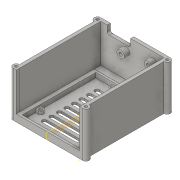
# Autodesk Inventor part: 11 electronics case
Saved by Autodesk Inventor 2016 (Build 200138000, 138)
## iProperties
Created: 2019-09-12
Part Number: 11 electronics case
Material: Generic
Document SubType Name: Modeling
Designer: mrbeh
Density: 1 g/cm^3
Appearance: Default
Author: mrbeh
Autodesk Inventor part; units mm, degrees
ref_plane "YZ Plane" through (0, 0, 0) normal (1, 0, 0) x (0, 1, 0)
ref_plane "XZ Plane" through (0, 0, 0) normal (0, 1, 0) x (-1, 0, 0)
ref_plane "XY Plane" through (0, 0, 0) normal (0, 0, 1) x (1, 0, 0)
sketch "Sketch1" plane through (0, 0, 0) normal (0, 1, 0) x (-1, 0, 0)
  line L0 (0, 0) -> (65, 0)
  line L1 (65, 0) -> (65, -85)
  line L2 (65, -85) -> (0, -85)
  line L3 (0, -85) -> (0, 0)
  dimension "d0" = 65
  dimension "d1" = 85
  constraints: 8 end point, 2 parallel, 1 horizontal, 1 perpendicular
  measures "d0" distance of L1.end L2.end
  measures "d1" distance of L0.end L1.end
extrude "Extrusion1" add sketch "Sketch1" along normal blind 2
sketch "Sketch2" plane through (0, 2, 0) normal (0, 1, 0) x (1, 0, 0)
  line L0 (-5.3227, 5.2279) -> (-58.5227, 5.2279)
  line L1 (-58.5227, 5.2279) -> (-58.5227, 73.9279)
  line L2 (-58.5227, 73.9279) -> (-5.3227, 73.9279)
  line L3 (-5.3227, 73.9279) -> (-5.3227, 5.2279)
  line L4 (-60.5227, 75.9279) -> (-60.5227, 3.2279)
  line L5 (-60.5227, 3.2279) -> (-3.3227, 3.2279)
  line L6 (-3.3227, 3.2279) -> (-3.3227, 75.9279)
  line L7 (-3.3227, 75.9279) -> (-60.5227, 75.9279)
  point P0 (0, 0)
  dimension "d4" = 53.2
  dimension "d5" = 68.7
  dimension "d6" = 2
  constraints: 16 end point, 4 parallel, 2 perpendicular, 1 horizontal, 3 other
  measures "d4" distance of L1.end L2.end
  measures "d5" distance of L0.end L1.end
  measures "d6" distance between parallel lines of L1 L4
extrude "Extrusion2" add sketch "Sketch2" along normal blind 5
ref_plane "Work Plane1" through (-31.9227, 2, -73.9279) normal (1, 0, 0) x (0, 0, -1)
sketch "Sketch4" plane through (0, 2, 0) normal (0, 1, 0) x (1, 0, 0)
  arc A0 (-56.0227, 17.7279) -> (-56.0227, 22.7279) centre (-56.0227, 20.2279) ccw
  line L0 (-58.5227, 5.2279) -> (-58.5227, 73.9279) projected
  line L1 (-56.0227, 17.7279) -> (-58.5227, 17.7279)
  line L2 (-58.5227, 17.7279) -> (-58.5227, 22.7279)
  line L3 (-58.5227, 22.7279) -> (-56.0227, 22.7279)
  point P0 (0, 0)
  dimension "d17" = 5
  constraints: 6 end point, 2 point on circle, 1 centre point, 1 horizontal, 1 parallel, 1 perpendicular, 1 point on line
  measures "d17" diameter of A0
extrude "Extrusion4" add sketch "Sketch4" along normal blind 3
sketch "Sketch5" plane through (0, 5, 0) normal (0, 1, 0) x (1, 0, 0)
  arc A0 (-56.0227, 17.7279) -> (-56.0227, 22.7279) centre (-56.0227, 20.2279) ccw projected
  circle A1 centre (-56.0227, 20.2279) radius 1.6
  point P0 (0, 0)
  dimension "d20" = 3.2
  constraints: 1 centre point, 1 coincident
  measures "d20" diameter of A1
extrude "Extrusion5" cut sketch "Sketch5" against normal blind 10
sketch "Sketch6" plane through (0, 2, 0) normal (0, 1, 0) x (1, 0, 0)
  line L0 (-5.3227, 73.9279) -> (-58.5227, 73.9279) projected
  line L1 (-5.3227, 73.9279) -> (-12.3227, 73.9279)
  line L2 (-5.3227, 71.4279) -> (-5.3227, 73.9279)
  arc A0 (-14.8227, 71.4279) -> (-9.8227, 71.4279) centre (-12.3227, 71.4279) ccw
  line L3 (-9.8227, 71.4279) -> (-9.8227, 73.9279)
  line L4 (-9.8227, 73.9279) -> (-14.8227, 73.9279)
  line L5 (-14.8227, 73.9279) -> (-14.8227, 71.4279)
  point P0 (0, 0)
  constraints: 10 end point, 2 point on circle, 1 centre point, 1 horizontal, 1 midpoint, 1 parallel, 1 point on line
extrude "Extrusion6" add sketch "Sketch6" along normal blind 3
sketch "Sketch7" plane through (0, 5, 0) normal (0, 1, 0) x (1, 0, 0)
  arc A0 (-14.8227, 71.4279) -> (-9.8227, 71.4279) centre (-12.3227, 71.4279) ccw projected
  circle A1 centre (-12.3227, 71.4279) radius 1.6
  point P0 (0, 0)
  dimension "d28" = 3.2
  constraints: 1 centre point, 1 coincident
  measures "d28" diameter of A1
extrude "Extrusion7" cut sketch "Sketch7" against normal blind 10
sketch "Sketch8" plane through (0, 2, 0) normal (0, 1, 0) x (1, 0, 0)
  line L0 (-5.3227, 5.2279) -> (-5.3227, 73.9279) projected
  line L1 (-5.3227, 73.9279) -> (-40.3227, 73.9279)
  line L2 (-5.3227, 71.4279) -> (-5.3227, 73.9279)
  arc A0 (-42.8227, 71.4279) -> (-37.8227, 71.4279) centre (-40.3227, 71.4279) ccw
  line L3 (-37.8227, 71.4279) -> (-37.8227, 73.9279)
  line L4 (-37.8227, 73.9279) -> (-42.8227, 73.9279)
  line L5 (-42.8227, 73.9279) -> (-42.8227, 71.4279)
  point P0 (0, 0)
  constraints: 10 end point, 2 point on circle, 1 centre point, 1 horizontal, 1 midpoint, 1 parallel, 1 point on line
extrude "Extrusion8" add sketch "Sketch8" along normal blind 3
sketch "Sketch9" plane through (0, 5, 0) normal (0, 1, 0) x (1, 0, 0)
  arc A0 (-42.8227, 71.4279) -> (-37.8227, 71.4279) centre (-40.3227, 71.4279) ccw projected
  circle A1 centre (-40.3227, 71.4279) radius 1.6
  point P0 (0, 0)
  dimension "d35" = 3.2
  constraints: 1 centre point, 1 coincident
  measures "d35" diameter of A1
extrude "Extrusion9" cut sketch "Sketch9" against normal blind 10
sketch "Sketch10" plane through (0, 2, 0) normal (0, 1, 0) x (1, 0, 0)
  line L0 (-5.3227, 5.2279) -> (-5.3227, 73.9279) projected
  line L1 (-5.3227, 19.2279) -> (-5.3227, 5.2279)
  arc A0 (-7.8227, 21.7279) -> (-7.8227, 16.7279) centre (-7.8227, 19.2279) ccw
  line L2 (-7.8227, 16.7279) -> (-5.3227, 16.7279)
  line L3 (-5.3227, 16.7279) -> (-5.3227, 21.7279)
  line L4 (-5.3227, 21.7279) -> (-7.8227, 21.7279)
  point P0 (0, 0)
  dimension "d40" = 5
  constraints: 8 end point, 2 point on circle, 1 centre point, 1 horizontal, 1 midpoint, 1 parallel, 1 perpendicular, 1 point on line
  measures "d40" diameter of A0
extrude "Extrusion10" add sketch "Sketch10" along normal blind 3
sketch "Sketch11" plane through (0, 5, 0) normal (0, 1, 0) x (1, 0, 0)
  arc A0 (-7.8227, 21.7279) -> (-7.8227, 16.7279) centre (-7.8227, 19.2279) ccw projected
  circle A1 centre (-7.8227, 19.2279) radius 1.6
  point P0 (0, 0)
  dimension "d43" = 3.2
  constraints: 1 centre point, 1 coincident
  measures "d43" diameter of A1
extrude "Extrusion11" cut sketch "Sketch11" against normal blind 10
sketch "Sketch12" plane through (0, 2, 0) normal (0, 1, 0) x (1, 0, 0)
  line L0 (-49.6328, 13.0575) -> (-14.6328, 13.0575)
  line L1 (-14.6328, 13.0575) -> (-14.6328, 17.0575)
  line L2 (-14.6328, 17.0575) -> (-49.6328, 17.0575)
  line L3 (-49.6328, 17.0575) -> (-49.6328, 13.0575)
  point P0 (0, 0)
  dimension "d46" = 35
  dimension "d47" = 4
  constraints: 8 end point, 2 parallel, 1 horizontal, 1 perpendicular
  measures "d46" distance of L2.end L1.end
  measures "d47" distance of L1.end L0.end
extrude "Extrusion12" cut sketch "Sketch12" against normal blind 10
fillet "Fillet1" radius 2 4 edges at (-49.6328, 1, -13.0575) (-49.6328, 1, -17.0575) (-14.6328, 1, -13.0575) (-14.6328, 1, -17.0575)
pattern_linear "Rectangular Pattern1" count 8 spacing 7 along (0, 0, -1) of "Extrusion12"
pattern_linear "Rectangular Pattern2" count 8 spacing 7 along (0, 0, -1) of "Fillet1"
sketch "Sketch13" plane through (0, 7, 0) normal (0, 1, 0) x (1, 0, 0)
  line L0 (4.8571, -9.3103) -> (-69.8772, -9.3103)
  line L1 (-69.8772, -9.3103) -> (-69.8772, 93.3248)
  line L2 (-69.8772, 93.3248) -> (4.8571, 93.3248)
  line L3 (4.8571, 93.3248) -> (4.8571, -9.3103)
  point P0 (0, 0)
  constraints: 8 end point, 2 parallel, 1 horizontal, 1 perpendicular
extrude "Extrusion13" cut sketch "Sketch13" against normal blind 0.5
sketch "Sketch14" plane through (0, 2, 0) normal (0, 1, 0) x (1, 0, 0)
  point P0 (0, 0)
sketch "Sketch15" plane through (0, 2, 0) normal (0, 1, 0) x (1, 0, 0)
  line L0 (0, 0) -> (-65, 0)
  line L1 (-65, 0) -> (-65, 3.228)
  line L2 (-65, 3.228) -> (0, 3.228)
  line L3 (0, 3.228) -> (0, 0)
  dimension "d59" = 65
  dimension "d60" = 3.228
  constraints: 8 end point, 2 parallel, 1 horizontal, 1 perpendicular
  measures "d59" distance of L1.end L2.end
  measures "d60" distance of L0.end L1.end
extrude "Extrusion14" cut sketch "Sketch15" against normal blind 5
sketch "Sketch18" plane through (0, 2, 0) normal (0, 1, 0) x (1, 0, 0)
  line L0 (0, 85) -> (-65, 85)
  line L1 (-65, 85) -> (-65, 82)
  line L2 (-65, 82) -> (0, 82)
  line L3 (0, 82) -> (0, 85)
  point P0 (0, 0)
  dimension "d63" = 65
  dimension "d64" = 3
  constraints: 8 end point, 2 parallel, 1 horizontal, 1 perpendicular
  measures "d63" distance of L2.end L1.end
  measures "d64" distance of L1.end L0.end
extrude "Extrusion15" add sketch "Sketch18" along normal blind 40
sketch "Sketch19" plane through (0, 2, 0) normal (0, 1, 0) x (1, 0, 0)
  line L0 (-65, 85) -> (0, 85) projected
  line L1 (-65, 3.228) -> (-62, 3.228)
  line L2 (-62, 3.228) -> (-62, 85)
  line L3 (-62, 85) -> (-65, 85)
  line L4 (-65, 85) -> (-65, 3.228)
  point P0 (0, 0)
  dimension "d67" = 3
  constraints: 8 end point, 2 parallel, 1 horizontal, 1 perpendicular, 1 point on line
  measures "d67" distance of L3.end L2.end
extrude "Extrusion16" add sketch "Sketch19" along normal blind 40
sketch "Sketch20" plane through (0, 2, 0) normal (0, 1, 0) x (1, 0, 0)
  line L0 (0, 3.228) -> (-65, 3.228) projected
  line L1 (-65, 85) -> (0, 85) projected
  line L2 (0, 3.228) -> (-3, 3.228)
  line L3 (-3, 3.228) -> (-3, 85)
  line L4 (-3, 85) -> (0, 85)
  line L5 (0, 85) -> (0, 3.228)
  point P0 (0, 0)
  dimension "d70" = 3
  constraints: 8 end point, 2 parallel, 1 horizontal, 1 perpendicular, 1 point on line
  measures "d70" distance of L3.end L4.end
extrude "Extrusion17" add sketch "Sketch20" along normal blind 40
sketch "Sketch21" plane through (0, 2, 0) normal (0, 1, 0) x (1, 0, 0)
  line L0 (-3.3227, 75.9279) -> (-3.3227, 3.2279) projected
  line L1 (-3, 82) -> (-3, 3.228) projected
  line L2 (-3.3227, 75.9279) -> (-3, 75.9279)
  line L3 (-3, 75.9279) -> (-3, 3.228)
  line L4 (-3, 3.228) -> (-3.3227, 3.228)
  line L5 (-3.3227, 3.228) -> (-3.3227, 75.9279)
  point P0 (0, 0)
  constraints: 8 end point, 2 parallel, 1 horizontal, 1 perpendicular
extrude "Extrusion18" add sketch "Sketch21" along normal blind 4.5
sketch "Sketch22" plane through (0, 2, 0) normal (0, 1, 0) x (1, 0, 0)
  line L0 (-62, 3.228) -> (-60.5227, 3.228) projected
  line L1 (-60.5227, 75.9279) -> (-62, 75.9279)
  line L2 (-62, 75.9279) -> (-62, 3.228)
  line L3 (-62, 3.228) -> (-60.5227, 3.228)
  line L4 (-60.5227, 3.228) -> (-60.5227, 75.9279)
  point P0 (0, 0)
  constraints: 8 end point, 2 parallel, 1 horizontal, 1 perpendicular
extrude "Extrusion19" add sketch "Sketch22" along normal blind 4.5
sketch "Sketch24" plane through (-60.5227, 6.5, -3.2279) normal (0, 0, 1) x (1, 0, 0)
  line L0 (-6.9309, 37.4653) -> (62.0283, 37.4653)
  line L1 (62.0283, 37.4653) -> (62.0283, -9.0596)
  line L2 (62.0283, -9.0596) -> (-6.9309, -9.0596)
  line L3 (-6.9309, -9.0596) -> (-6.9309, 37.4653)
  point P0 (60.5227, -6.5)
  constraints: 8 end point, 2 parallel, 1 horizontal, 1 perpendicular
extrude "Extrusion20" cut sketch "Sketch24" against normal blind 0.01
sketch "Sketch25" plane through (-62, 2, -82) normal (0, 0, 1) x (1, 0, 0)
  circle A0 centre (49.0531, 31.4134) radius 3.5
  point P0 (62, -2)
  dimension "d79" = 7
  constraints: 1 centre point
  measures "d79" diameter of A0
extrude "Extrusion21" add sketch "Sketch25" along normal blind 5
sketch "Sketch26" plane through (-62, 2, -82) normal (0, 0, 1) x (1, 0, 0)
  circle A0 centre (49.0531, 31.4134) radius 3.5 projected
  circle A1 centre (23.5531, 27.7134) radius 3.5
  point P0 (62, -2)
  dimension "d84" = 7
  constraints: 1 centre point
  measures "d84" diameter of A1
extrude "Extrusion22" add sketch "Sketch26" along normal blind 5 contours A1
sketch "Sketch27" plane through (-62, 2, -82) normal (0, 0, 1) x (1, 0, 0)
  line L0 (0, 40) -> (59, 40) projected
  line L1 (27.8808, 40) -> (6.0561, 40)
  line L2 (6.0561, 40) -> (6.0561, 32.7591)
  line L3 (6.0561, 32.7591) -> (27.8808, 32.7591)
  line L4 (27.8808, 32.7591) -> (27.8808, 40)
  point P0 (62, -2)
  constraints: 8 end point, 2 parallel, 1 horizontal, 1 perpendicular, 1 point on line
extrude "Extrusion23" cut sketch "Sketch27" against normal blind 5
fillet "Fillet2" radius 2 2 edges at (-55.9439, 34.7591, -83.5) (-34.1192, 34.7591, -83.5)
sketch "Sketch28" plane through (-38.4469, 29.7134, -77) normal (0, 0, 1) x (1, 0, 0)
  circle A0 centre (0, 0) radius 1.6
  point P0 (38.4469, -29.7134)
  dimension "d90" = 3.2
  constraints: 1 centre point
  measures "d90" diameter of A0
extrude "Extrusion24" cut sketch "Sketch28" against normal blind 10
sketch "Sketch30" plane through (0, 2, 0) normal (0, 1, 0) x (1, 0, 0)
  line L0 (-3, 82) -> (-62, 82) projected
  line L1 (-62, 82) -> (-3, 82)
  line L2 (-3, 82) -> (-3, 75.9718)
  line L3 (-3, 75.9718) -> (-62, 75.9718)
  line L4 (-62, 75.9718) -> (-62, 82)
  point P0 (0, 0)
  constraints: 8 end point, 2 parallel, 1 horizontal, 1 perpendicular
extrude "Extrusion25" add sketch "Sketch30" along normal blind 4.5
sketch "Sketch31" plane through (-12.9469, 33.4134, -77) normal (0, 0, 1) x (1, 0, 0)
  circle A0 centre (0, 0) radius 1.6
  point P0 (12.9469, -33.4134)
  dimension "d95" = 3.2
  constraints: 1 centre point
  measures "d95" diameter of A0
extrude "Extrusion26" cut sketch "Sketch31" against normal blind 10
sketch "Sketch32" plane through (0, 42, 0) normal (0, 1, 0) x (1, 0, 0)
  line L0 (0, 85) -> (0, 3.2379) projected
  circle A0 centre (0, 6.238) radius 3.0001
  point P0 (0, 0)
  constraints: 1 point on line, 1 vertical alignment, 2 other
extrude "Extrusion27" add sketch "Sketch32" against normal blind 42
pattern_linear "Rectangular Pattern3" count 2 spacing 75.762 along (0, 0, -1) count 2 spacing 65 along (-1, 0, 0) of "Extrusion27"
sketch "Sketch33" plane through (0, 42, 0) normal (0, 1, 0) x (1, 0, 0)
  arc A0 (0, 3.2379) -> (0, 9.2381) centre (0, 6.238) ccw projected
  circle A1 centre (0, 6.238) radius 1.25
  point P0 (0, 0)
  dimension "d106" = 2.5
  constraints: 1 centre point, 1 coincident
  measures "d106" diameter of A1
extrude "Extrusion28" cut sketch "Sketch33" against normal blind 42
pattern_linear "Rectangular Pattern4" count 2 spacing 75.762 along (0, 0, -1) count 2 spacing 65 along (-1, 0, 0) of "Extrusion28"
body "Solid1"
